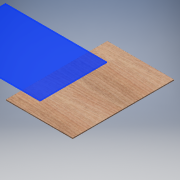
# Autodesk Inventor part: Electronics plate
Saved by Autodesk Inventor 2019.4 (Build 234330000, 330)
## iProperties
Created: 2019-12-08
Part Number: Electronics plate
Material: Wood (Birch)
Document SubType Name: Modeling
Designer: admin
Density: 0.55 g/cm^3
Appearance: Birch - Natural Polished
Mass: 243.54 g
Surface Area: 2268.4 cm^2
Volume: 442.8 cm^3
Author: admin
Autodesk Inventor part; units mm, degrees
ref_plane "YZ Plane" through (0, 0, 0) normal (1, 0, 0) x (0, 1, 0)
ref_plane "XZ Plane" through (0, 0, 0) normal (0, 1, 0) x (-1, 0, 0)
ref_plane "XY Plane" through (0, 0, 0) normal (0, 0, 1) x (1, 0, 0)
sketch "Sketch1" plane through (0, 0, 0) normal (0, 1, 0) x (-1, 0, 0)
  line L0 (-135, 205) -> (135, 205)
  line L1 (135, 205) -> (135, -205)
  line L2 (135, -205) -> (-135, -205)
  line L3 (-135, -205) -> (-135, 205)
  line L4 (-135, 205) -> (135, -205) construction
  line L5 (135, 205) -> (-135, -205) construction
  point P0 (0, 0)
  dimension "d0" = 270
  dimension "d1" = 410
  constraints: 12 end point, 2 midpoint, 2 parallel, 1 horizontal, 1 perpendicular
  measures "d0" distance of L1.end L2.end
  measures "d1" distance of L0.end L1.end
extrude "Extrusion1" add sketch "Sketch1" along normal blind 4
body "Solid1"
